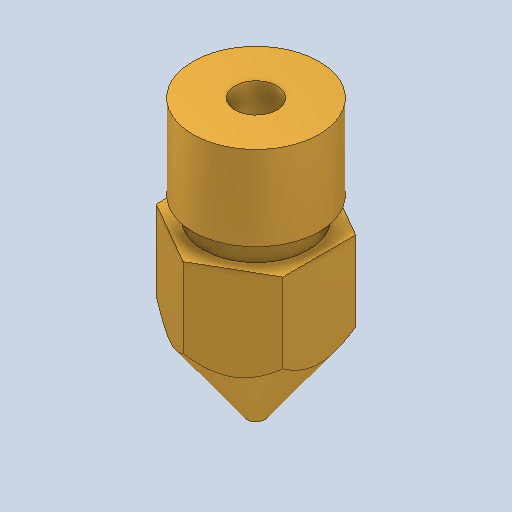
# Autodesk Inventor part: ENDER 3 NOZZLE
Saved by Autodesk Inventor 2022 (Build 260153070, 153G)
## iProperties
Created: 2022-01-01
Part Number: ENDER 3 NOZZLE
Material: Brass, Soft Yellow
Document SubType Name: Modeling
Designer: a laptop
Density: 8.47 g/cm^3
Appearance: Brass - Satin
Author: a laptop
Autodesk Inventor part; units mm, degrees
ref_plane "YZ Plane" through (0, 0, 0) normal (1, 0, 0) x (0, 1, 0)
ref_plane "XZ Plane" through (0, 0, 0) normal (0, 1, 0) x (-1, 0, 0)
ref_plane "XY Plane" through (0, 0, 0) normal (0, 0, 1) x (1, 0, 0)
sketch "Sketch1" plane through (0, 0, 0) normal (0, 0, 1) x (1, 0, 0)
  line L0 (-3, 13) -> (-3, 9)
  line L1 (-3, 9) -> (-2.5, 9)
  line L2 (-2.5, 9) -> (-2.5, 8)
  line L3 (-0.45, 0) -> (0, 0)
  line L4 (0, 0) -> (0, 13) construction
  line L5 (-1, 13) -> (-1, 1.6)
  line L6 (-1, 1.6) -> (-0.2, 0.8)
  line L7 (-0.2, 0.8) -> (-0.2, 0)
  line L8 (-1, 13) -> (-3, 13)
  line L9 (-3.7774, 8) -> (-3.7774, 4.6648)
  line L10 (-3.7774, 4.6648) -> (-0.45, 0)
  line L11 (-2.5, 8) -> (-3.7774, 8)
  dimension "d0" = 3
  dimension "d1" = 13
  dimension "d2" = 9
  dimension "d5" = 0.45
  dimension "d6" = 2.5
  dimension "d7" = 45
  dimension "d8" = 1
  dimension "d9" = 0.2
  dimension "d10" = 0.8
  dimension "d12" = 3.5774
  dimension "d13" = 8
  dimension "d14" = 35.5
  constraints: 24 end point, 8 perpendicular, 1 coincident, 1 horizontal, 1 horizontal alignment, 1 parallel, 1 point on line
  measures "d0" distance of L4.end L0.start
  measures "d1" vertical distance of point (0, 0) L0.start
  measures "d2" vertical distance of point (0, 0) L0.end
  measures "d5" distance of L3.start L3.end
  measures "d6" distance from line of point (0, 0) L2
  measures "d7" angle of L4 L6
  measures "d8" distance from line of point (0, 0) L5
  measures "d9" distance of point (0, 0) L7.end
  measures "d10" vertical distance of point (0, 0) L6.end
  measures "d12" horizontal distance of L7.end L9.start
  measures "d13" vertical distance of L7.end L9.start
  measures "d14" angle of L4 L10
revolve "Revolution1" add sketch "Sketch1" angle 360 about axis through (0, 0, 0) along (0, 1, 0)
sketch "Sketch2" plane through (0, 0, 0) normal (0, -1, 0) x (1, 0, 0)
  line L0 (3, -1.7321) -> (0, -3.4641)
  line L1 (0, -3.4641) -> (-3, -1.7321)
  line L2 (-3, -1.7321) -> (-3, 1.7321)
  line L3 (-3, 1.7321) -> (0, 3.4641)
  line L4 (0, 3.4641) -> (3, 1.7321)
  line L5 (3, 1.7321) -> (3, -1.7321)
  circle A0 centre (0, 0) radius 5
  circle A1 centre (0, 0) radius 0.45 construction
  point P0 (0, 0)
  dimension "d15" = 6
  dimension "d17" = 10
  constraints: 12 end point, 1 centre point, 1 coincident, 1 concentric, 1 vertical, 13 other
  measures "d15" distance between parallel lines of L2 L5
  measures "d17" diameter of A0
extrude "Extrusion1" cut sketch "Sketch2" against normal blind 8
body "Solid1"
